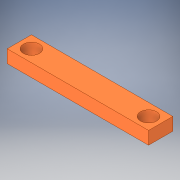
# Autodesk Inventor part: Pinza_acople
Saved by Autodesk Inventor 2019 (Build 230136000, 136)
## iProperties
Created: 2020-02-07
Part Number: Pinza_acople
Material: Generic
Document SubType Name: Modeling
Designer: Omar
Density: 1 g/cm^3
Appearance: Default
Author: Omar
Autodesk Inventor part; units mm, degrees
ref_plane "YZ Plane" through (0, 0, 0) normal (1, 0, 0) x (0, 1, 0)
ref_plane "XZ Plane" through (0, 0, 0) normal (0, 1, 0) x (-1, 0, 0)
ref_plane "XY Plane" through (0, 0, 0) normal (0, 0, 1) x (1, 0, 0)
sketch "Sketch1" plane through (0, 0, 0) normal (0, 1, 0) x (-1, 0, 0)
  line L0 (0, 0) -> (35, 0)
  line L1 (35, 0) -> (35, -6)
  line L2 (35, -6) -> (0, -6)
  line L3 (0, -6) -> (0, 0)
  circle A0 centre (32, -3) radius 2
  circle A1 centre (3, -3) radius 2
  dimension "d0" = 35
  dimension "d1" = 6
  dimension "d2" = 4
  dimension "d3" = 4
  dimension "d4" = 3
  dimension "d5" = 3
  dimension "d6" = 3
  dimension "d7" = 3
  constraints: 8 end point, 2 centre point, 2 parallel, 1 horizontal, 1 perpendicular
  measures "d0" distance of L1.end L2.end
  measures "d1" distance of L0.end L1.end
  measures "d2" diameter of A0
  measures "d3" diameter of A1
  measures "d4" distance from line of L0 A0.centre
  measures "d5" distance from line of L1 A0.centre
  measures "d6" distance from line of L3 A1.centre
  measures "d7" distance from line of L0 A1.centre
extrude "Extrusion1" add sketch "Sketch1" along normal blind 3.18
body "Solid1"
